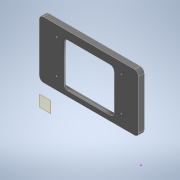
# Autodesk Inventor part: Ventilator Screen Arm 01
Saved by Autodesk Inventor 2021 (Build 250183000, 183)
## iProperties
Created: 2020-04-14
Part Number: Ventilator Screen Arm 01
Material: PAEK Plastic
Document SubType Name: Modeling
Designer: James
Density: 1.32 g/cm^3
Appearance: Gray
Author: James
Autodesk Inventor part; units mm, degrees
ref_plane "Work Plane5" through (-196, 0, 0) normal (0, 0, 1) x (1, 0, 0)
sketch "Sketch13" plane through (-196, 0, 0) normal (0, 0, 1) x (1, 0, 0)
  line L0 (7.5, 44.9846) -> (184.5156, 44.9846)
  line L1 (192.5, 52.4846) -> (192.5, 147.9846)
  line L2 (184.5, 155.9846) -> (7.5, 155.9846)
  line L3 (-0.5, 147.9846) -> (-0.5, 52.9846)
  arc A0 (-0.5, 52.9846) -> (7.5, 44.9846) centre (7.5, 52.9846) ccw
  arc A1 (184.5156, 44.9846) -> (192.5, 52.4846) centre (184.5156, 52.9846) ccw
  arc A2 (7.5, 155.9846) -> (-0.5, 147.9846) centre (7.5, 147.9846) ccw
  arc A3 (192.5, 147.9846) -> (184.5, 155.9846) centre (184.5, 147.9846) ccw
  line L4 (6.5, 147.9846) -> (6.5, 52.9846)
  arc A4 (6.5, 52.9846) -> (7.5, 51.9846) centre (7.5, 52.9846) ccw
  line L5 (7.5, 51.9846) -> (184.5156, 51.9846)
  arc A5 (184.5156, 51.9846) -> (185.5, 52.8084) centre (184.5156, 52.9846) ccw
  line L6 (185.5, 52.8084) -> (185.5, 147.9846)
  arc A6 (185.5, 147.9846) -> (184.5, 148.9846) centre (184.5, 147.9846) ccw
  line L7 (184.5, 148.9846) -> (7.5, 148.9846)
  arc A7 (7.5, 148.9846) -> (6.5, 147.9846) centre (7.5, 147.9846) ccw
  point P0 (-0.5, 44.9846)
  point P1 (192.5, 155.9846)
  point P2 (192.5, 44.9846)
  point P3 (-0.5, 155.9846)
  dimension "d79" = 8
  dimension "d112" = 8
  dimension "d117" = 7
  constraints: 16 end point, 16 point on circle, 8 centre point, 8 point on line, 7 tangent, 2 equal radius, 2 parallel, 1 horizontal, 7 other
  measures "d79" radius of A0
  measures "d112" radius of A2
  measures "d117" radial gap between concentric circles of A2 A7
extrude "Extrusion9" add sketch "Sketch13" along normal blind 11.1
ref_plane "Work Plane6" through (-196, 0, 0) normal (0, 0, -1) x (-1, 0, 0)
sketch "Sketch14" plane through (-196, 0, 0) normal (0, 0, -1) x (-1, 0, 0)
  line L0 (-144.7002, 132.1649) -> (-144.7002, 67.5846)
  line L1 (-47.7002, 67.5846) -> (-47.7002, 132.5846)
  line L2 (-55.2002, 140.0846) -> (-137.2002, 140.0846)
  line L3 (-144.7002, 132.5846) -> (-144.7002, 132.1649)
  arc A0 (-137.2002, 140.0846) -> (-144.7002, 132.5846) centre (-137.2002, 132.5846) ccw
  arc A1 (-47.7002, 132.5846) -> (-55.2002, 140.0846) centre (-55.2002, 132.5846) ccw
  line L4 (-192.5, 100.2346) -> (-248.457, 100.2346)
  line L5 (-96, 155.9846) -> (-96, 209.6502)
  line L6 (-47.7002, 67.5846) -> (-47.7002, 62.4846)
  line L7 (-144.7002, 67.5846) -> (-144.7002, 62.4846)
  line L8 (-137.2002, 54.9846) -> (-55.2002, 54.9846)
  arc A2 (-55.2002, 54.9846) -> (-47.7002, 62.4846) centre (-55.2002, 62.4846) ccw
  arc A3 (-144.7002, 62.4846) -> (-137.2002, 54.9846) centre (-137.2002, 62.4846) ccw
  line L9 (-184.5, 155.9846) -> (-7.5, 155.9846) projected
  line L10 (-192.5, 52.4846) -> (-192.5, 147.9846) projected
  line L11 (0.5, 147.9846) -> (0.5, 52.9846) projected
  line L12 (0.5, 147.9846) -> (0.5, 163.3157)
  line L13 (0.5, 163.3157) -> (-33.72, 163.3157)
  circle A4 centre (-159, 134.6846) radius 1.25
  line L14 (-159, 134.6846) -> (-159, 68.6846)
  circle A5 centre (-159, 68.6846) radius 1.25
  line L15 (-159, 68.6846) -> (-33, 68.6846)
  circle A6 centre (-33, 68.6846) radius 1.25
  line L16 (-33, 68.6846) -> (-33, 134.6846)
  circle A7 centre (-33, 134.6846) radius 1.25
  line L17 (-184.5156, 51.9846) -> (-7.5, 51.9846) projected
  point P0 (-196, 0)
  point P1 (-181.3, 148.9846)
  point P2 (-13.3, 148.9846)
  point P3 (-47.7002, 140.0846)
  point P4 (-144.7002, 140.0846)
  dimension "d80" = 97
  dimension "d83" = 7.5
  dimension "d111" = 7.5
  dimension "d126" = 34.22
  dimension "d132" = 2.5
  dimension "d133" = 33.5
  dimension "d134" = 21.3
  dimension "d135" = 66
  dimension "d136" = 2.5
  dimension "d138" = 126
  dimension "d139" = 2.5
  dimension "d140" = 2.5
  dimension "d142" = 3
  constraints: 28 end point, 8 centre point, 8 point on circle, 8 tangent, 8 vertical, 5 point on line, 4 perpendicular, 3 coincident, 2 equal radius, 2 horizontal
  measures "d80" distance of point (-47.7, 140.085) point (-144.7, 140.085)
  measures "d83" radius of A0
  measures "d111" radius of A2
  measures "d126" distance of L12.end L13.end
  measures "d132" diameter of A4
  measures "d133" distance from line of L10 L14.start
  measures "d134" distance from line of L9 L14.start
  measures "d135" distance of L14.start L14.end
  measures "d136" diameter of A5
  measures "d138" distance of L15.start L15.end
  measures "d139" diameter of A6
  measures "d140" diameter of A7
  measures "d142" distance between parallel lines of L17 L8
ref_plane "Work Plane3" through (-196, 0, 0) normal (0, 0, -1) x (-1, 0, 0)
sketch "Sketch16" plane through (-196, 0, 0) normal (0, 0, -1) x (-1, 0, 0)
  line L0 (-181.3, 148.9846) -> (-6.5, 148.9846)
  line L1 (-6.5, 148.9846) -> (-6.5, 47)
  line L2 (-6.5, 47) -> (-181.3, 47)
  line L3 (-6.5, 52.9846) -> (-6.5, 147.9846) projected
  line L4 (-185.5, 147.9846) -> (-185.5, 52.8084) projected
  line L5 (-181.3, 47) -> (-185.5, 47)
  line L6 (-185.5, 47) -> (-185.5, 148.9846)
  line L7 (-185.5, 148.9846) -> (-6.5, 148.9846)
  line L8 (-6.5, 148.9846) -> (-185.5, 148.9846)
  point P0 (-196, 0)
  constraints: 14 end point, 3 perpendicular, 2 equal length, 2 horizontal
extrude "Extrusion11" add sketch "Sketch16" against normal up to surface (11.1 mm away)
extrude "Extrusion12" cut sketch "Sketch14" against normal up to surface (11.1 mm away)
ref_plane "Work Plane2" through (-196, 0, 10) normal (0, 0, 1) x (1, 0, 0)
sketch "Sketch18" plane through (-196, 0, 10) normal (0, 0, 1) x (1, 0, 0)
  point P0 (196, 0)
extrude "Extrusion14" cut sketch "Sketch13" along normal blind 8 contours A7 L7 A6 L6 A5 L5 A4 L4
body "Solid1"
